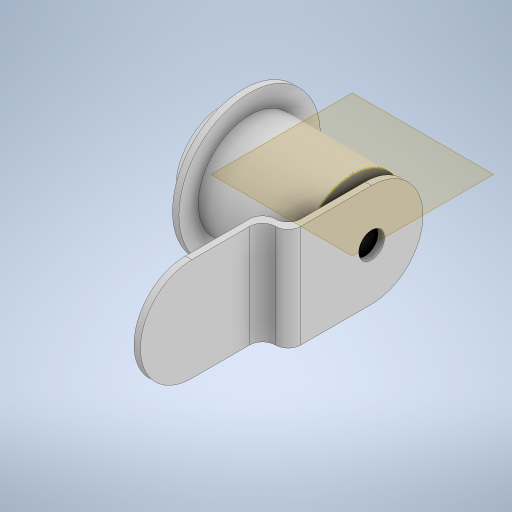
# Autodesk Inventor part: Замок
Saved by Autodesk Inventor 2023 (Build 270158000, 158)
## iProperties
Created: 2022-04-27
Part Number: Замок
Material: Типовые
Document SubType Name: Modeling
Designer: User
Density: 1 g/cm^3
Appearance: По умолчанию
Author: User
Autodesk Inventor part; units mm, degrees
ref_plane "YZ Plane" through (0, 0, 0) normal (1, 0, 0) x (0, 1, 0)
ref_plane "XZ Plane" through (0, 0, 0) normal (0, 1, 0) x (-1, 0, 0)
ref_plane "XY Plane" through (0, 0, 0) normal (0, 0, 1) x (1, 0, 0)
sketch "Эскиз1" plane through (0, 0, 0) normal (0, 1, 0) x (-1, 0, 0)
  line L0 (0, 0) -> (0, -8)
  line L1 (0, -8) -> (16, -8)
  line L2 (16, -8) -> (16, -11)
  line L3 (16, -11) -> (17, -11)
  line L4 (17, 0) -> (20, 0)
  line L5 (20, 0) -> (20, -7.5)
  line L6 (20, -7.5) -> (17, -11)
  line L7 (0, 0) -> (17, 0)
  dimension "d0" = 8
  dimension "d1" = 16
  dimension "d2" = 3
  dimension "d3" = 1
  dimension "d4" = 3
  dimension "d5" = 7.5
  constraints: 16 end point, 3 perpendicular, 1 horizontal, 1 vertical
  measures "d0" distance of L0.start L0.end
  measures "d1" distance of L0.end L1.end
  measures "d2" distance of L1.end L2.end
  measures "d3" distance of L2.end L3.end
  measures "d4" distance of L4.start L4.end
  measures "d5" distance of L4.end L5.end
revolve "Вращение1" add sketch "Эскиз1" angle 360 about axis through (0, 0, 0) along (-1, 0, 0)
sketch "Эскиз2" plane through (0, 0, 0) normal (1, 0, 0) x (0, 0, -1)
  circle A0 centre (0, 0) radius 8 projected
  point P0 (0, 8)
  constraints: 1 vertical alignment, 1 other
ref_plane "РабПлоскость1" through (0, 8, 0) normal (0, 1, 0) x (-1, 0, 0)
sketch "Эскиз3" plane through (0, 8, 0) normal (0, 1, 0) x (-1, 0, 0)
  line L0 (0, -8) -> (16, -8) projected
  line L1 (0, -8) -> (-1, -8)
  line L2 (-1, -8) -> (-2, -8)
  line L3 (-2, -8) -> (-2, 12)
  line L4 (-2, 12) -> (2, 12)
  line L5 (2, 12) -> (2, 32)
  line L6 (2, 32) -> (1, 32)
  line L7 (1, 32) -> (1, 14)
  line L8 (1, 14) -> (1, 13)
  line L9 (1, 13) -> (-3, 13)
  line L10 (-3, 13) -> (-3, -8)
  line L11 (-3, -8) -> (-2, -8)
  point P0 (0, 0)
  dimension "d7" = 1
  dimension "d8" = 1
  dimension "d9" = 20
  dimension "d10" = 4
  dimension "d11" = 20
  dimension "d12" = 1
  dimension "d13" = 18
  dimension "d14" = 1
  dimension "d15" = 4
  constraints: 22 end point, 8 perpendicular, 4 point on line, 1 collinear
  measures "d7" distance of L1.start L1.end
  measures "d8" distance of L1.end L2.end
  measures "d9" distance of L2.end L3.end
  measures "d10" distance of L3.end L4.end
  measures "d11" distance of L4.end L5.end
  measures "d12" distance of L5.end L6.end
  measures "d13" distance of L6.end L7.end
  measures "d14" distance of L7.end L8.end
  measures "d15" distance of L8.end L9.end
extrude "Выдавливание1" add sketch "Эскиз3" against normal blind 16
fillet "Сопряжение1" radius 2 2 edges at (-1, 0, 13) (3, 0, 13)
fillet "Сопряжение2" radius 2 2 edges at (-2, 0, 12) (2, 0, 12)
fillet "Сопряжение3" radius 8 4 edges at (2.5, 8, -8) (2.5, -8, -8) (-1.5, 8, 32) (-1.5, -8, 32)
sketch "Эскиз4" plane through (3, -8, 11) normal (1, 0, 0) x (0, 0, -1)
  circle A0 centre (11, 8) radius 2
  dimension "d21" = 4
  constraints: 1 centre point, 1 coincident
  measures "d21" diameter of A0
extrude "Выдавливание2" cut sketch "Эскиз4" against normal blind 8
sketch "Эскиз5" plane through (-20, 0, 0) normal (-1, 0, 0) x (0, 0, 1)
  line L0 (0, 0) -> (4, 0)
  line L1 (4, 0) -> (4, 1)
  line L2 (4, 1) -> (-4, 1)
  line L3 (-4, 1) -> (-4, -1)
  line L4 (-4, -1) -> (4, -1)
  line L5 (4, -1) -> (4, 0)
  dimension "d24" = 4
  dimension "d25" = 1
  dimension "d26" = 8
  dimension "d27" = 2
  constraints: 12 end point, 5 perpendicular, 1 horizontal, 1 point on line
  measures "d24" distance of L0.start L0.end
  measures "d25" distance of L0.end L1.end
  measures "d26" distance of L1.end L2.end
  measures "d27" distance of L2.end L3.end
extrude "Выдавливание3" cut sketch "Эскиз5" against normal blind 7
